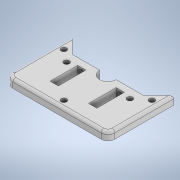
# Autodesk Inventor part: g2HEMount1
Saved by Autodesk Inventor 2020 (Build 240168000, 168)
## iProperties
Created: 2021-06-01
Part Number: g2HEMount1
Material: Generic
Document SubType Name: Modeling
Designer: PAB
Density: 1 g/cm^3
Appearance: Default
Author: PAB
Autodesk Inventor part; units mm, degrees
ref_plane "YZ Plane" through (0, 0, 0) normal (1, 0, 0) x (0, 1, 0)
ref_plane "XZ Plane" through (0, 0, 0) normal (0, 1, 0) x (-1, 0, 0)
ref_plane "XY Plane" through (0, 0, 0) normal (0, 0, 1) x (1, 0, 0)
sketch "Sketch1" plane through (0, 0, 0) normal (0, 1, 0) x (-1, 0, 0)
  line L0 (37, 37) -> (-37, 37)
  line L1 (-37, 37) -> (-37, -37)
  line L2 (-37, -37) -> (37, -37)
  line L3 (37, -37) -> (37, 37)
  point P0 (0, 0)
  dimension "d0" = 74
  dimension "d1" = 74
  constraints: 8 end point, 2 parallel, 1 horizontal, 1 perpendicular
  measures "d0" distance of L2.end L1.end
  measures "d1" distance of L1.end L0.end
extrude "Extrusion1" add sketch "Sketch1" along normal blind 6
fillet "Fillet1" radius 5 4 edges at (-37, 3, 37) (37, 3, 37) (37, 3, -37) (-37, 3, -37)
sketch "Sketch2" plane through (0, 6, 0) normal (0, 1, 0) x (1, 0, 0)
  line L0 (-37, 32) -> (-37, -32) projected
  line L1 (-37, 0) -> (37, 0)
  line L2 (37, -32) -> (37, 32) projected
  circle A0 centre (0, 0) radius 6
  line L3 (-37, 0) -> (37, 0)
  line L4 (37, 0) -> (37, 63.5)
  line L5 (37, 63.5) -> (-37, 63.5)
  line L6 (-37, 63.5) -> (-37, 0)
  line L7 (-6, 0) -> (-26, 0)
  line L8 (-26, 0) -> (-37, 11)
  line L9 (6, 0) -> (26, 0)
  line L10 (26, 0) -> (37, 11)
  circle A1 centre (32, 0) radius 2
  circle A2 centre (0, -32) radius 2
  circle A3 centre (-32, 0) radius 2
  point P0 (-6, 0)
  dimension "d5" = 12
  dimension "d6" = 20
  dimension "d7" = 135
  dimension "d8" = 20
  dimension "d9" = 135
  dimension "d10" = 4
  dimension "d11" = 4
  dimension "d12" = 4
  constraints: 18 end point, 8 point on line, 4 centre point, 2 midpoint, 2 parallel, 2 point on circle, 1 coincident, 1 horizontal, 1 perpendicular
  measures "d5" diameter of A0
  measures "d6" distance of L7.start L7.end
  measures "d7" angle of L7 L8
  measures "d8" distance of L9.start L9.end
  measures "d9" angle of L10 L9
  measures "d10" diameter of A1
  measures "d11" diameter of A2
  measures "d12" diameter of A3
extrude "Extrusion2" cut sketch "Sketch2" against normal blind 10 contours L6 L5 L4 L2 L10 L1 A0 L8 L0 | A3 L1 | L1 A3 | A0 L1 | L1 A0 | A1 L1 | L1 A1 | A2
sketch "Sketch3" plane through (0, 6, 0) normal (0, 1, 0) x (1, 0, 0)
  line L0 (11, -5) -> (17, -5)
  line L1 (17, -5) -> (17, -25)
  line L2 (17, -25) -> (11, -25)
  line L3 (11, -25) -> (11, -5)
  line L4 (-11, -5) -> (-17, -5)
  line L5 (-17, -5) -> (-17, -25)
  line L6 (-17, -25) -> (-11, -25)
  line L7 (-11, -25) -> (-11, -5)
  point P0 (0, 0)
  dimension "d15" = 6
  dimension "d16" = 20
  dimension "d17" = 6
  constraints: 16 end point, 4 parallel, 2 horizontal, 2 perpendicular, 1 point on line
  measures "d15" distance of L1.end L2.end
  measures "d16" distance of L0.end L1.end
  measures "d17" distance of L6.end L5.end
extrude "Extrusion3" cut sketch "Sketch3" against normal blind 10
sketch "Sketch4" plane through (26, 6, 0) normal (0, 0, -1) x (-1, 0, 0)
  circle A0 centre (12, -3) radius 2
  circle A1 centre (40, -3) radius 2
  point P0 (26, -6)
  dimension "d20" = 4
  dimension "d21" = 4
  constraints: 2 centre point
  measures "d20" diameter of A0
  measures "d21" diameter of A1
extrude "Extrusion4" cut sketch "Sketch4" against normal blind 10
fillet "Fillet2" radius 2 5 edges at (35.5355, 6, 35.5355) (0, 6, 37) (-35.5355, 6, 35.5355) (-37, 6, 10.5) (37, 6, 10.5)
sketch "Sketch5" plane through (0, 6, 0) normal (0, 1, 0) x (1, 0, 0)
  circle A0 centre (23, -7) radius 2
  circle A1 centre (-23, -7) radius 2
  point P0 (0, 0)
  dimension "d25" = 4
  dimension "d26" = 4
  constraints: 2 centre point
  measures "d25" diameter of A0
  measures "d26" diameter of A1
extrude "Extrusion5" cut sketch "Sketch5" against normal blind 10
body "Solid1"
